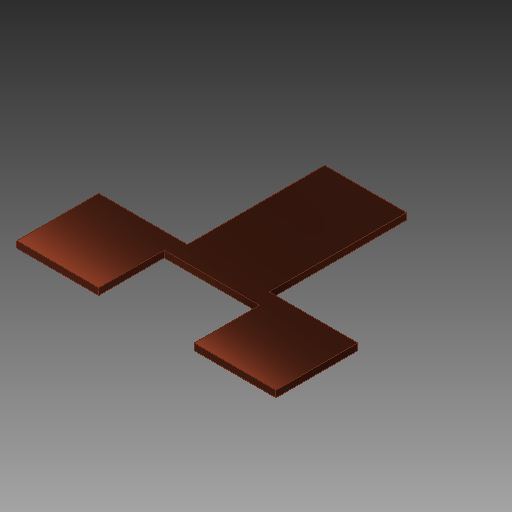
# Autodesk Inventor part: Copper Plate
Saved by Autodesk Inventor 2019.2 (Build 232265000, 265)
## iProperties
Created: 2018-12-13
Part Number: Copper Plate
Material: Copper
Document SubType Name: Modeling
Designer: Petar
Density: 8.94 g/cm^3
Appearance: Copper - Polished
Author: Petar
Autodesk Inventor part; units mm, degrees
ref_plane "YZ Plane" through (0, 0, 0) normal (1, 0, 0) x (0, 1, 0)
ref_plane "XZ Plane" through (0, 0, 0) normal (0, 1, 0) x (-1, 0, 0)
ref_plane "XY Plane" through (0, 0, 0) normal (0, 0, 1) x (1, 0, 0)
derived "Housing Box 1.ipt"
sketch "Sketch19" plane through (-44.5974, 65.8623, 31.5139) normal (0, 1, 0) x (1, 0, 0)
  line L0 (0, 0) -> (0, -106.9722)
  line L1 (89.1948, 0) -> (89.1948, -106.9722)
  line L2 (84.1948, -101.9722) -> (84.1948, -76.9722)
  line L3 (5, -76.9722) -> (5, -101.9722)
  line L4 (57.0974, -76.9722) -> (57.0974, -35)
  line L5 (57.0974, -35) -> (32.0974, -35)
  line L6 (32.0974, -35) -> (32.0974, -76.9722)
  line L7 (84.1948, -76.9722) -> (57.0974, -76.9722)
  line L8 (32.0974, -76.9722) -> (5, -76.9722)
  line L9 (59.1948, -101.9722) -> (59.1948, -81.9722)
  line L10 (59.1948, -81.9722) -> (30, -81.9722)
  line L11 (30, -81.9722) -> (30, -101.9722)
  line L12 (5, -101.9722) -> (30, -101.9722)
  line L13 (59.1948, -101.9722) -> (84.1948, -101.9722)
  line L14 (89.1948, 0) -> (0, 0)
  line L15 (0, -106.9722) -> (89.1948, -106.9722)
  line L16 (44.5974, -106.9722) -> (44.5974, 0) construction
  line L17 (6, -100.9722) -> (29, -100.9722)
  line L18 (29, -100.9722) -> (29, -77.9722)
  line L19 (29, -77.9722) -> (6, -77.9722)
  line L20 (6, -77.9722) -> (6, -100.9722)
  line L21 (83.1948, -77.9722) -> (83.1948, -100.9722)
  line L22 (83.1948, -100.9722) -> (60.1948, -100.9722)
  line L23 (60.1948, -100.9722) -> (60.1948, -77.9722)
  line L24 (60.1948, -77.9722) -> (83.1948, -77.9722)
  point P0 (44.5974, 31.5139)
extrude "Extrusion1" add sketch "Sketch19" along normal blind 2 contours L13 L9 L10 L11 L12 L3 L8 L6 L5 L4 L7 L2 | L20 L19 L18 L17 | L21 L22 L23 L24
body "Solid1"
